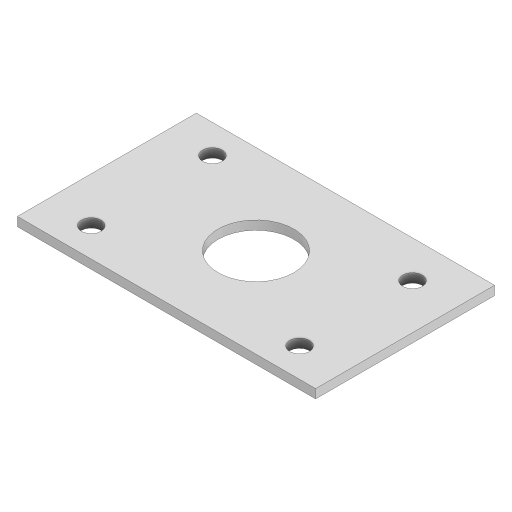
# Autodesk Inventor part: Base V6
Saved by Autodesk Inventor 2024.1 (Build 281209000, 209)
## iProperties
Created: 2023-11-30
Part Number: Base V6
Material: Generic
Document SubType Name: Modeling
Designer: dbt5238
Density: 1 g/cm^3
Appearance: Default
Author: dbt5238
Autodesk Inventor part; units mm, degrees
ref_plane "YZ Plane" through (0, 0, 0) normal (1, 0, 0) x (0, 1, 0)
ref_plane "XZ Plane" through (0, 0, 0) normal (0, 1, 0) x (-1, 0, 0)
ref_plane "XY Plane" through (0, 0, 0) normal (0, 0, 1) x (1, 0, 0)
sketch "Sketch1" plane through (0, 0, 0) normal (0, 1, 0) x (-1, 0, 0)
  line L0 (50, 30) -> (-50, 30)
  line L1 (-50, 30) -> (-50, -30)
  line L2 (-50, -30) -> (50, -30)
  line L3 (50, -30) -> (50, 30)
  line L4 (50, 30) -> (-50, -30) construction
  line L5 (-50, 30) -> (50, -30) construction
  point P0 (0, 0)
  dimension "d0" = 100
  dimension "d1" = 60
  constraints: 12 end point, 2 midpoint, 2 parallel, 1 horizontal, 1 perpendicular
  measures "d0" distance of L1.end L2.end
  measures "d1" distance of L2.end L0.start
extrude "Extrusion1" add sketch "Sketch1" along normal blind 3
sketch "Sketch2" plane through (0, 3, 0) normal (0, 1, 0) x (1, 0, 0)
  point P0 (0, 0)
  point P1 (-34.925, 20.32)
  point P2 (-34.925, -20.32)
  point P3 (34.925, -20.32)
  point P4 (34.925, 17.5675)
  dimension "d11" = 69.85
  dimension "d12" = 34.925
  dimension "d13" = 40.64
  dimension "d15" = 20.32
  constraints: 2 vertical alignment, 1 horizontal alignment
  measures "d11" horizontal distance of point (34.925, 17.568) point (-34.925, 20.32)
  measures "d12" horizontal distance of point (0, 0) point (-34.925, 20.32)
  measures "d13" distance of point (-34.925, -20.32) point (-34.925, 20.32)
  measures "d15" vertical distance of point (-34.925, 20.32) point (0, 0)
hole "Hole1" at (-34.925, 3, -20.32) at (-34.925, 3, 20.32) at (34.925, 3, 20.32) at (34.925, 3, -17.5675) direction (0, -1, 0) diameter 6.6 end through all clearance for "Hex Head Bolt" size "M6" standard "Ansi Metric M Profile"
sketch "Sketch3" plane through (0, 3, 0) normal (0, 1, 0) x (1, 0, 0)
  circle A0 centre (0, 0) radius 12.7
  dimension "d16" = 25.4
  constraints: 1 centre point, 1 coincident
  measures "d16" diameter of A0
extrude "Extrusion2" cut sketch "Sketch3" against normal through all
equation "\"d12\" = 0.5 * d11"
equation "\"d15\" = 0.5 * d13"
body "Solid1"
